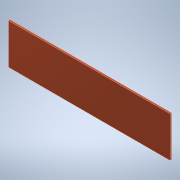
# Autodesk Inventor part: 8005_Cu_groundplane_Tx_Filter_Stage1_MPSv2_v1
Saved by Autodesk Inventor 2021 (Build 250183000, 183)
## iProperties
Created: 2021-04-07
Part Number: 8005_Cu_groundplane_Tx_Filter_Stage1_MPSv2_v1
Material: Copper
Document SubType Name: Modeling
Designer: Barksdale
Density: 8.94 g/cm^3
Appearance: Copper - Satin
Author: Barksdale
Autodesk Inventor part; units mm, degrees
ref_plane "YZ Plane" through (0, 0, 0) normal (1, 0, 0) x (0, 1, 0)
ref_plane "XZ Plane" through (0, 0, 0) normal (0, 1, 0) x (-1, 0, 0)
ref_plane "XY Plane" through (0, 0, 0) normal (0, 0, 1) x (1, 0, 0)
sketch "Sketch1" plane through (0, 0, 0) normal (0, 0, 1) x (1, 0, 0)
  line L0 (-11.7086, 5.9971) -> (88.2914, 5.9971)
  line L1 (88.2914, 5.9971) -> (88.2914, -19.0029)
  line L2 (88.2914, -19.0029) -> (-11.7086, -19.0029)
  line L3 (-11.7086, -19.0029) -> (-11.7086, 5.9971)
  point P0 (0, 0)
  dimension "d0" = 100
  dimension "d1" = 25
  constraints: 8 end point, 2 parallel, 1 horizontal, 1 perpendicular
  measures "d0" distance of L1.end L2.end
  measures "d1" distance of L0.end L1.end
extrude "Extrusion1" add sketch "Sketch1" along normal blind 1
body "Solid1"
